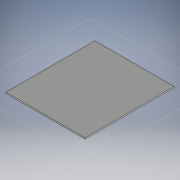
# Autodesk Inventor part: 000.001.014 - Грузовая площадка
Saved by Autodesk Inventor 2022 (Build 260153000, 153)
## iProperties
Created: 2023-06-09
Part Number: 000.001.014 - Грузовая площадка
Material: Типовые
Document SubType Name: Modeling
Designer: Иван Петров
Density: 1 g/cm^3
Appearance: По умолчанию
Author: Иван Петров
Autodesk Inventor part; units mm, degrees
ref_plane "YZ Plane" through (0, 0, 0) normal (1, 0, 0) x (0, 1, 0)
ref_plane "XZ Plane" through (0, 0, 0) normal (0, 1, 0) x (-1, 0, 0)
ref_plane "XY Plane" through (0, 0, 0) normal (0, 0, 1) x (1, 0, 0)
sketch "Эскиз1" plane through (0, 0, 0) normal (0, 1, 0) x (-1, 0, 0)
  line L0 (-128, 144) -> (128, 144)
  line L1 (128, 144) -> (128, -144)
  line L2 (128, -144) -> (-128, -144)
  line L3 (-128, -144) -> (-128, 144)
  line L4 (-128, 144) -> (128, -144) construction
  line L5 (128, 144) -> (-128, -144) construction
  point P0 (0, 0)
  dimension "d0" = 256
  dimension "d1" = 288
  constraints: 12 end point, 2 midpoint, 2 parallel, 1 horizontal, 1 perpendicular
  measures "d0" distance of L1.end L2.end
  measures "d1" distance of L0.end L1.end
extrude "Выдавливание1" add sketch "Эскиз1" along normal blind 4
sketch "Эскиз2" plane through (0, 0, 0) normal (0, -1, 0) x (1, 0, 0)
  circle A0 centre (-26, 81.25) radius 2 projected
  circle A1 centre (-26, -81.25) radius 2 projected
  circle A2 centre (-112, 56) radius 1.85 projected
  circle A3 centre (-112, -56) radius 1.85 projected
  circle A4 centre (120, 128) radius 1.85 projected
  circle A5 centre (112, 120) radius 1.85 projected
  circle A6 centre (104, 128) radius 1.85 projected
  circle A7 centre (112, 136) radius 1.85 projected
  circle A8 centre (-112, 136) radius 1.85 projected
  circle A9 centre (-104, 128) radius 1.85 projected
  circle A10 centre (-112, 120) radius 1.85 projected
  circle A11 centre (-120, 128) radius 1.85 projected
  circle A12 centre (-104, -128) radius 1.85 projected
  circle A13 centre (-120, -128) radius 1.85 projected
  circle A14 centre (-112, -120) radius 1.85 projected
  circle A15 centre (-112, -136) radius 1.85 projected
  circle A16 centre (104, -128) radius 1.85 projected
  circle A17 centre (112, -120) radius 1.85 projected
  circle A18 centre (112, -136) radius 1.85 projected
  circle A19 centre (120, -128) radius 1.85 projected
  point P0 (0, 0)
extrude "Выдавливание2" cut sketch "Эскиз2" against normal blind 4
